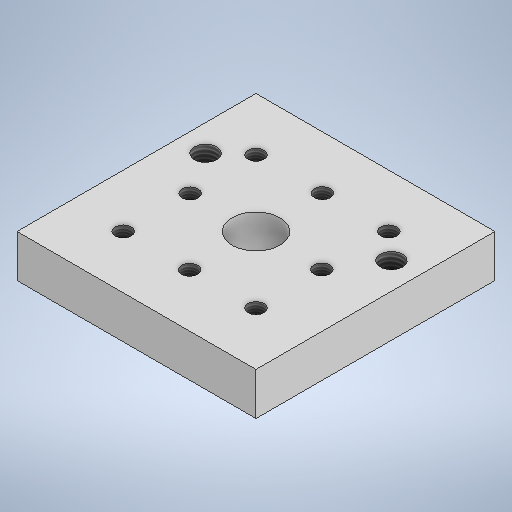
# Autodesk Inventor part: liftmotorfloor
Saved by Autodesk Inventor 2025.2 (Build 292293000, 293)
## iProperties
Created: 2026-03-22
Part Number: liftmotorfloor
Material: Generic
Document SubType Name: Modeling
Designer: hp
Density: 1 g/cm^3
Appearance: Default
Author: hp
Autodesk Inventor part; units mm, degrees
ref_plane "YZ Plane" through (0, 0, 0) normal (1, 0, 0) x (0, 1, 0)
ref_plane "XZ Plane" through (0, 0, 0) normal (0, 1, 0) x (-1, 0, 0)
ref_plane "XY Plane" through (0, 0, 0) normal (0, 0, 1) x (1, 0, 0)
sketch "Sketch1" plane through (0, 0, 0) normal (0, 1, 0) x (-1, 0, 0)
  circle A0 centre (-1.4813, 2.0187) radius 4.5
  circle A1 centre (16.0187, -5.9813) radius 2.1
  circle A2 centre (-18.9813, -5.9813) radius 2.1
  arc A3 (-18.9813, -2.4813) -> (-18.9813, -9.4813) centre (-18.9813, -5.9813) ccw
  arc A4 (16.0187, -9.4813) -> (16.0187, -2.4813) centre (16.0187, -5.9813) ccw
  line L0 (8.5187, -7.9813) -> (-11.4813, -7.9813)
  line L1 (-11.4813, -7.9813) -> (-11.4813, 12.0187)
  line L2 (-11.4813, 12.0187) -> (8.5187, 12.0187)
  line L3 (8.5187, 12.0187) -> (8.5187, -7.9813)
  line L4 (8.5187, -7.9813) -> (-11.4813, 12.0187) construction
  line L5 (-11.4813, -7.9813) -> (8.5187, 12.0187) construction
  line L6 (-16.4813, 17.0187) -> (13.5187, 17.0187)
  line L7 (13.5187, 17.0187) -> (13.5187, -12.9813)
  line L8 (13.5187, -12.9813) -> (-16.4813, -12.9813)
  line L9 (-16.4813, -12.9813) -> (-16.4813, 17.0187)
  line L10 (-16.4813, 17.0187) -> (13.5187, -12.9813) construction
  line L11 (13.5187, 17.0187) -> (-16.4813, -12.9813) construction
  circle A5 centre (10.9187, 2.0187) radius 1.5
  circle A6 centre (-1.4813, 14.5187) radius 1.5
  circle A7 centre (-1.4813, -10.4813) radius 1.5
  circle A8 centre (11.0187, -10.4813) radius 1.5
  circle A9 centre (11.0187, 14.5187) radius 1.5
  line L12 (-1.4813, -12.9813) -> (-1.4813, 17.0187)
  circle A10 centre (-13.9813, -10.4813) radius 1.5
  circle A11 centre (-13.8813, 2.0187) radius 1.5
  circle A12 centre (-13.9813, 14.5187) radius 1.5
  line L13 (-23.9813, 24.5187) -> (21.0187, 24.5187)
  line L14 (21.0187, 24.5187) -> (21.0187, -20.4813)
  line L15 (21.0187, -20.4813) -> (-23.9813, -20.4813)
  line L16 (-23.9813, -20.4813) -> (-23.9813, 24.5187)
  line L17 (-23.9813, 24.5187) -> (21.0187, -20.4813) construction
  line L18 (21.0187, 24.5187) -> (-23.9813, -20.4813) construction
  point P0 (0, 0)
  point P1 (-1.4813, -5.9813)
  point P2 (-1.4813, 2.0187)
  point P3 (8.5187, 2.0187)
  dimension "d0" = 20
  dimension "d1" = 20
  dimension "d2" = 30
  dimension "d3" = 30
  dimension "d4" = 3
  dimension "d5" = 3
  dimension "d6" = 3
  dimension "d7" = 12.5
  dimension "d8" = 12.4
  dimension "d9" = 12.5
  dimension "d10" = 3
  dimension "d11" = 3
  dimension "d12" = 12.5
  dimension "d13" = 45
  dimension "d14" = 45
  constraints: 38 end point, 13 centre point, 9 midpoint, 6 parallel, 4 point on circle, 3 horizontal, 3 perpendicular, 3 symmetric about line, 2 point on line, 3 other
  measures "d0" distance of L4.end L5.end
  measures "d1" distance of L5.start L4.end
  measures "d2" distance of L10.end L11.end
  measures "d3" distance of L6.end L10.end
  measures "d4" diameter of A5
  measures "d5" diameter of A6
  measures "d6" diameter of A7
  measures "d7" distance of point (-1.481, 2.019) A7.centre
  measures "d8" distance of point (-1.481, 2.019) A5.centre
  measures "d9" distance of point (-1.481, 2.019) A6.centre
  measures "d10" diameter of A8
  measures "d11" diameter of A9
  measures "d12" horizontal distance of point (-1.481, 2.019) A9.centre
  measures "d13" distance of L14.end L15.end
  measures "d14" distance of L13.end L14.end
extrude "Extrusion1" add sketch "Sketch1" against normal blind 8 contours A0 L12 L2 L3 L0 | A0 L12 L0 L1 L2 | L12 A6 L6 L7 L8 A7 L0 L3 L2 | L2 L1 L0 L12 A7 L8 L9 L6 A6 | L13 L14 L15 L16
thread "Thread1" size "M4.5x0.75" class "6H" standard "ISO Metric profile" length 8
thread "Thread2" size "M4.5x0.75" class "6H" standard "ISO Metric profile" length 8
thread "Thread3" size "M3x0.5" class "6H" standard "ISO Metric profile" length 8
thread "Thread4" size "M3x0.5" class "6H" standard "ISO Metric profile" length 8
thread "Thread5" size "M3x0.5" class "6H" standard "ANSI Metric M Profile" length 8
thread "Thread6" size "M3x0.5" class "6H" standard "ISO Metric profile" length 8
thread "Thread7" size "M3x0.5" class "6H" standard "ISO Metric profile" length 8
thread "Thread8" size "M3x0.5" class "6H" standard "ISO Metric profile" length 8
thread "Thread9" size "M3x0.5" class "6H" standard "ISO Metric profile" length 8
thread "Thread10" size "M3x0.5" class "6H" standard "ISO Metric profile" length 8
body "Solid1"
